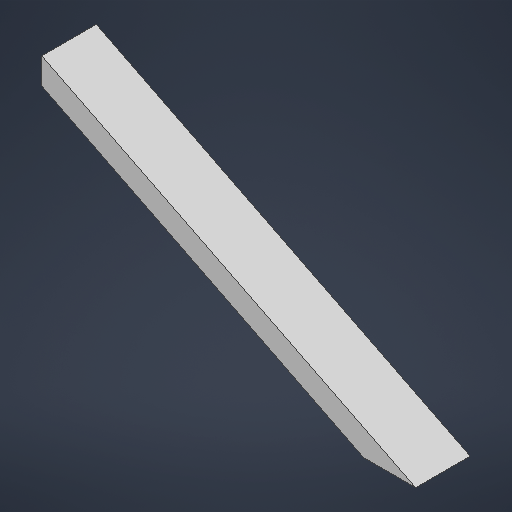
# Autodesk Inventor part: S2_2x4x26.833
Saved by Autodesk Inventor 2026 (Build 300175000, 175)
## iProperties
Created: 2025-09-03
Part Number: S2_2x4x26.833
Material: Generic
Document SubType Name: Modeling
Designer: trott
Density: 1 g/cm^3
Appearance: Default
Author: trott
Autodesk Inventor part; units mm, degrees
ref_plane "YZ Plane" through (0, 0, 0) normal (1, 0, 0) x (0, 1, 0)
ref_plane "XZ Plane" through (0, 0, 0) normal (0, 1, 0) x (-1, 0, 0)
ref_plane "XY Plane" through (0, 0, 0) normal (0, 0, 1) x (1, 0, 0)
sketch "Sketch1" plane through (0, 0, 0) normal (0, 0, 1) x (1, 0, 0)
  line L0 (0, 0) -> (0, 304.8)
  line L1 (0, 0) -> (609.6, 0)
  line L2 (0, 304.8) -> (609.6, 0)
  line L3 (609.6, 0) -> (592.5612, -34.0777)
  line L4 (0, 304.8) -> (-17.0388, 270.7223)
  line L5 (-17.0388, 270.7223) -> (592.5612, -34.0777)
  point P0 (0, 262.2029)
  point P1 (524.4058, 0)
  dimension "d1" = 304.8
  dimension "d2" = 609.6
  dimension "d3" = 38.1
  dimension "d4" = 38.1
  dimension "d5" = 90
  constraints: 12 end point, 1 horizontal, 1 perpendicular, 1 vertical
  measures "d1" distance of L0.start L0.end
  measures "d2" distance of L0.start L1.end
  measures "d3" distance of L1.end L3.end
  measures "d4" distance of L0.end L4.end
  measures "d5" angle of L2 L4
extrude "Extrusion1" add sketch "Sketch1" along normal blind 88.9 contours L0 L2 L1 L5
body "Solid1"
